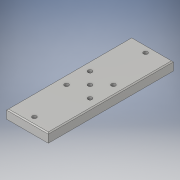
# Autodesk Inventor part: Platform A
Saved by Autodesk Inventor 2019.4 (Build 234330000, 330)
## iProperties
Created: 2021-01-08
Part Number: Platform A
Material: Generic
Document SubType Name: Modeling
Designer: caleb
Density: 1 g/cm^3
Appearance: Default
Author: caleb
Autodesk Inventor part; units mm, degrees
ref_plane "YZ Plane" through (0, 0, 0) normal (1, 0, 0) x (0, 1, 0)
ref_plane "XZ Plane" through (0, 0, 0) normal (0, 1, 0) x (-1, 0, 0)
ref_plane "XY Plane" through (0, 0, 0) normal (0, 0, 1) x (1, 0, 0)
sketch "Sketch1" plane through (0, 0, 0) normal (0, 1, 0) x (-1, 0, 0)
  line L0 (-14.9987, 44.9961) -> (14.9987, 44.9961)
  line L1 (14.9987, 44.9961) -> (14.9987, -44.9961)
  line L2 (14.9987, -44.9961) -> (-14.9987, -44.9961)
  line L3 (-14.9987, -44.9961) -> (-14.9987, 44.9961)
  line L4 (-14.9987, 44.9961) -> (14.9987, -44.9961) construction
  line L5 (14.9987, 44.9961) -> (-14.9987, -44.9961) construction
  point P0 (0, 0)
  dimension "d0" = 89.9922
  dimension "d1" = 29.9974
  constraints: 12 end point, 2 midpoint, 2 parallel, 1 horizontal, 1 perpendicular
  measures "d0" distance of L0.end L1.end
  measures "d1" distance of L0.start L0.end
extrude "Extrusion1" add sketch "Sketch1" along normal blind 6.35
sketch "Sketch2" plane through (0, 6.35, 0) normal (0, 1, 0) x (1, 0, 0)
  circle A0 centre (-8.4201, -8.4201) radius 1.4986
  line L0 (-14.9987, 44.9961) -> (-14.9987, -44.9961) projected
  line L1 (-14.9987, -44.9961) -> (14.9987, -44.9961) projected
  circle A1 centre (-8.4201, 8.4201) radius 1.4986
  circle A2 centre (8.4201, -8.4201) radius 1.4986
  circle A3 centre (8.4201, 8.4201) radius 1.4986
  point P0 (0, 0)
  dimension "d4" = 2.9972
  dimension "d5" = 8.4201
  dimension "d8" = 16.8402
  dimension "d11" = 16.8402
  dimension "d14" = 8.4201
  constraints: 4 centre point, 1 horizontal, 1 vertical, 6 other
  measures "d4" diameter of A0
  measures "d5" horizontal distance of A0.centre point (0, 0)
  measures "d8" distance of A0.centre A1.centre
  measures "d11" distance of A0.centre A2.centre
  measures "d14" horizontal distance of point (0, 0) A0.centre
hole "Hole1" at (8.4201, 6.35, -8.4201) at (-8.4201, 6.35, -8.4201) at (-8.4201, 6.35, 8.4201) at (8.4201, 6.35, 8.4201) direction (0, -1, 0) diameter 2.9972 end through all
sketch "Sketch3" plane through (0, 6.35, 0) normal (0, 1, 0) x (1, 0, 0)
  circle A0 centre (0, 0) radius 1.4986
  dimension "d22" = 2.9972
  constraints: 1 centre point, 1 coincident
  measures "d22" diameter of A0
extrude "Extrusion2" cut sketch "Sketch3" against normal through all
sketch "Sketch4" plane through (0, 0, 0) normal (0, -1, 0) x (1, 0, 0)
  line L0 (-4.0005, 35.0012) -> (4.0005, 35.0012)
  line L1 (4.0005, 35.0012) -> (4.0005, -35.0012)
  line L2 (4.0005, -35.0012) -> (-4.0005, -35.0012)
  line L3 (-4.0005, -35.0012) -> (-4.0005, 35.0012)
  line L4 (-4.0005, 35.0012) -> (4.0005, -35.0012) construction
  line L5 (4.0005, 35.0012) -> (-4.0005, -35.0012) construction
  point P0 (0, 0)
  dimension "d25" = 8.001
  dimension "d26" = 70.0024
  constraints: 12 end point, 2 midpoint, 2 parallel, 1 horizontal, 1 perpendicular
  measures "d25" distance of L1.end L2.end
  measures "d26" distance of L0.end L1.end
extrude "Extrusion3" cut sketch "Sketch4" against normal blind 1.4986
fillet "Fillet1" radius 2.032 4 edges at (4.0005, 0.7493, 35.0012) (-4.0005, 0.7493, 35.0012) (-4.0005, 0.7493, -35.0012) (4.0005, 0.7493, -35.0012)
sketch "Sketch5" plane through (0, 6.35, 0) normal (0, 1, 0) x (1, 0, 0)
  circle A0 centre (0, -39.9923) radius 1.4986
  circle A1 centre (0, 39.9923) radius 1.4986
  line L0 (-14.9987, -44.9961) -> (14.9987, -44.9961) projected
  line L1 (14.9987, 44.9961) -> (-14.9987, 44.9961) projected
  point P0 (0, 0)
  dimension "d33" = 2.9972
  dimension "d34" = 2.9972
  dimension "d35" = 5.0038
  dimension "d36" = 5.0038
  constraints: 2 centre point
  measures "d33" diameter of A0
  measures "d34" diameter of A1
  measures "d35" distance from line of L0 A0.centre
  measures "d36" distance from line of L1 A1.centre
extrude "Extrusion4" cut sketch "Sketch5" against normal through all
chamfer "Chamfer2" distance 0.7112 angle 45 4 edges at (14.9987, 6.35, 0) (0, 6.35, 44.9961) (-14.9987, 6.35, 0) (0, 6.35, -44.9961)
body "Solid1"
